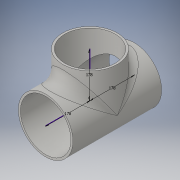
# Autodesk Inventor part: 8in tee sch40
Saved by Autodesk Inventor 2016 (Build 200138000, 138)
## iProperties
Created: 2016-08-28
Part Number: 8in tee sch40
Material: Generic
Document SubType Name: Modeling
Designer: Luiz Henrique
Density: 1 g/cm^3
Appearance: Default
Author: Luiz Henrique
Autodesk Inventor part; units mm, degrees
ref_plane "YZ Plane" through (0, 0, 0) normal (1, 0, 0) x (0, 1, 0)
ref_plane "XZ Plane" through (0, 0, 0) normal (0, 1, 0) x (-1, 0, 0)
ref_plane "XY Plane" through (0, 0, 0) normal (0, 0, 1) x (1, 0, 0)
sketch "Sketch1" plane through (0, 0, 0) normal (1, 0, 0) x (0, 1, 0)
  line L0 (0, 0) -> (0, 178)
  line L1 (0, 0) -> (0, -178)
  line L2 (0, 0) -> (178, 0)
  dimension "d0" = 178
  dimension "d1" = 178
  dimension "d2" = 178
  constraints: 6 end point, 2 vertical, 1 horizontal
  measures "d0" distance of L0.start L0.end
  measures "d1" distance of L0.start L1.end
  measures "d2" distance of L0.start L2.end
sketch "Sketch2" plane through (0, 0, 0) normal (0, 0, 1) x (1, 0, 0)
  circle A0 centre (0, 0) radius 109.5
  circle A1 centre (0, 0) radius 101.32
  dimension "d3" = 219
  dimension "d4" = 8.18
  constraints: 2 centre point, 1 coincident
  measures "d3" diameter of A0
  measures "d4" radial gap between concentric circles of A0 A1
sketch "Sketch3" plane through (0, 0, 0) normal (0, 1, 0) x (-1, 0, 0)
  circle A0 centre (0, 0) radius 109.5
  circle A1 centre (0, 0) radius 101.32
  dimension "d5" = 219
  dimension "d6" = 8.18
  constraints: 2 centre point, 1 coincident
  measures "d5" diameter of A0
  measures "d6" radial gap between concentric circles of A0 A1
extrude "Extrusion1" add sketch "Sketch2" along normal mid plane 356
extrude "Extrusion2" add sketch "Sketch3" along normal blind 178
sketch "Sketch4" plane through (0, 0, 178) normal (0, 0, 1) x (1, 0, 0)
  circle A0 centre (0, 0) radius 101.32
  constraints: 1 centre point, 1 coincident
extrude "Extrusion3" cut sketch "Sketch4" against normal blind 500
sketch "Sketch5" plane through (0, 178, 0) normal (0, 1, 0) x (1, 0, 0)
  circle A0 centre (0, 0) radius 101.32
  constraints: 1 centre point, 1 coincident
extrude "Extrusion4" cut sketch "Sketch5" against normal blind 178
fillet "Fillet1" radius 50 2 edges at (0, 109.5, 109.5) (0, 109.5, -109.5)
body "Solid1"
